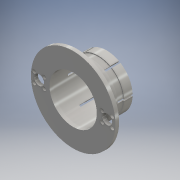
# Autodesk Inventor part: Fixture
Saved by Autodesk Inventor 2016 (Build 200138000, 138)
## iProperties
Created: 2015-07-19
Part Number: Fixture
Material: Generic
Document SubType Name: Modeling
Designer: bastli
Density: 1 g/cm^3
Appearance: Aluminum - Polished
Author: bastli
Autodesk Inventor part; units mm, degrees
ref_plane "YZ Plane" through (0, 0, 0) normal (1, 0, 0) x (0, 1, 0)
ref_plane "XZ Plane" through (0, 0, 0) normal (0, 1, 0) x (-1, 0, 0)
ref_plane "XY Plane" through (0, 0, 0) normal (0, 0, 1) x (1, 0, 0)
sketch "Sketch1" plane through (0, 0, 0) normal (0, 1, 0) x (-1, 0, 0)
  circle A0 centre (0, 0) radius 67.77
  circle A1 centre (0, 0) radius 38.45
  circle A2 centre (0, 0) radius 41.45
  circle A3 centre (0, 0) radius 37.95
  line L0 (67.77, 0) -> (-67.77, 0) construction
  line L1 (0, 67.77) -> (0, -67.77) construction
  line L2 (62.61, -8) -> (46.61, -8) construction
  line L3 (46.61, -8) -> (46.61, 8) construction
  line L4 (46.61, 8) -> (62.61, 8) construction
  line L5 (62.61, 8) -> (62.61, -8) construction
  line L6 (62.61, -8) -> (46.61, 8) construction
  line L7 (46.61, -8) -> (62.61, 8) construction
  line L8 (64.77, -10.16) -> (44.45, -10.16) construction
  line L9 (44.45, -10.16) -> (44.45, 10.16) construction
  line L10 (44.45, 10.16) -> (64.77, 10.16) construction
  line L11 (64.77, 10.16) -> (64.77, -10.16) construction
  line L12 (64.77, -10.16) -> (44.45, 10.16) construction
  line L13 (44.45, -10.16) -> (64.77, 10.16) construction
  line L14 (64.77, 0) -> (67.77, 0) construction
  line L15 (44.45, 0) -> (41.45, 0) construction
  circle A4 centre (54.61, 0) radius 7.995
  circle A5 centre (-54.61, 0) radius 7.995
  point P0 (-62.61, 8)
  point P1 (-46.61, 8)
  point P2 (-46.61, -8)
  point P3 (-62.61, -8)
  dimension "d0" = 135.54
  dimension "d1" = 76.9
  dimension "d2" = 3
  dimension "d3" = 75.9
  dimension "d4" = 16
  dimension "d5" = 16
  dimension "d6" = 20.32
  dimension "d7" = 20.32
  dimension "d30" = 15.99
  constraints: 32 end point, 9 midpoint, 8 coincident, 5 centre point, 5 symmetric about line, 4 parallel, 4 point on circle, 3 horizontal, 2 collinear, 2 perpendicular, 2 point on line, 1 horizontal alignment, 1 vertical, 3 other
  measures "d0" diameter of A0
  measures "d1" diameter of A1
  measures "d3" diameter of A3
  measures "d4" distance of L3.end L4.end
  measures "d5" distance of L4.end L2.start
  measures "d6" distance of L9.end L10.end
  measures "d7" distance of L10.end L8.start
  measures "d30" diameter of A4
extrude "Extrusion1" add sketch "Sketch1" against normal blind 6 contours A0 | A1 | A2 | A4 | A5
extrude "Extrusion2" add sketch "Sketch1" along normal blind 48 contours A2
ref_plane "Work Plane1" through (0, 24, 0) normal (0, 1, 0) x (1, 0, 0)
sketch "Sketch2" plane through (0, 24, 0) normal (0, 1, 0) x (1, 0, 0)
  circle A0 centre (0, 0) radius 38.45 projected
  circle A1 centre (0, 0) radius 41.45 projected
  circle A2 centre (0, 0) radius 39.95
  dimension "d14" = 1.5
  constraints: 1 centre point
  measures "d14" radial gap between concentric circles of A1 A2
extrude "Extrusion3" cut sketch "Sketch2" along normal blind 10 contours A1
sketch "Sketch3" plane through (0, 48, 0) normal (0, 1, 0) x (1, 0, 0)
  circle A0 centre (0, 0) radius 41.45 projected
  circle A1 centre (0, 0) radius 38.45 projected
  line L0 (0, 0) -> (41.45, 0) construction
  line L1 (0, 0) -> (41.4247, 1.4466) construction
  circle A2 centre (0, 0) radius 41.45 projected
  line L2 (0, 0) -> (41.4247, -1.4466) construction
  line L3 (41.4247, 1.4466) -> (38.4266, 1.3419)
  circle A3 centre (0, 0) radius 38.45 projected
  line L4 (41.4247, -1.4466) -> (38.4266, -1.3419)
  dimension "d17" = 4
  constraints: 10 end point, 7 point on circle, 2 point on line, 1 horizontal, 1 other
  measures "d17" angle of L2 L1
extrude "Extrusion4" cut sketch "Sketch3" against normal up to surface (24 mm away) contours A0 L4 A1 L3 picked at (40.4482, -0.3099)
pattern_circular "Circular Pattern1" count 6 over 360 about axis through (0, 0, 0) along (0, 1, 0) of "Extrusion4"
fillet "Fillet1" radius 3 1 edges at (41.45, 0, 0)
hole "Hole1" at (-62.61, 0, 8) at (-46.61, 0, 8) at (-46.61, 0, -8) at (-62.61, 0, -8) at (62.61, 0, 8) at (46.61, 0, 8) at (46.61, 0, -8) at (62.61, 0, -8) direction (0, -1, 0) diameter 3.4 end through all
extrude "Extrusion5" cut sketch "Sketch1" against normal through all contours A4 | A5
sketch "Sketch4" plane through (0, -6, 0) normal (0, -1, 0) x (1, 0, 0)
  circle A0 centre (-46.61, -8) radius 1.7 construction
  circle A1 centre (-62.61, 8) radius 1.7 construction
  circle A2 centre (-46.61, 8) radius 1.7 construction
  circle A3 centre (46.61, 8) radius 1.7 construction
  circle A4 centre (46.61, -8) radius 1.7 construction
  circle A5 centre (62.61, -8) radius 1.7 construction
  circle A6 centre (62.61, 8) radius 1.7 construction
  circle A7 centre (-62.61, -8) radius 1.7 construction
  point P0 (0, 0)
  constraints: 8 coincident
hole "Hole2" at (-62.61, -6, 8) at (-46.61, -6, 8) at (-46.61, -6, -8) at (-62.61, -6, -8) at (46.61, -6, -8) at (46.61, -6, 8) at (62.61, -6, 8) at (62.61, -6, -8) direction (0, 1, 0) diameter 6 depth 3 tip angle 118
equation "\"d0\" = outer_radius"
equation "\"d1\" = pvc_radius"
equation "\"d2\" = thickness"
equation "\"d3\" = pcv_foot_radius"
equation "\"d4\" = nema_8_hole_distance"
equation "\"d5\" = nema_8_hole_distance"
equation "\"d6\" = nema_8_width"
equation "\"d7\" = nema_8_width"
equation "\"d8\" = 2 * thickness"
equation "\"d10\" = fixture_height"
equation "\"d14\" = 0.5 * thickness"
equation "\"d33\" = m3_head"
equation "\"d38\" = thickness"
equation "\"thickness\" = 3"
equation "\"outer_radius\" = 6 * thickness + pvc_radius + 2 * nema_8_width"
equation "\"pvc_radius\" = 76.9"
equation "\"pcv_foot_radius\" = 75.9"
equation "\"nema_8_width\" = 20.32"
equation "\"nema_8_hole_distance\" = 16"
equation "\"fixture_height\" = 16 * thickness"
equation "\"d13\" = 0.5 * fixture_height"
equation "\"m3_through\" = 3.4"
equation "\"m3_head\" = 6"
equation "\"m3_hold\" = 3.1"
body "Solid1"
